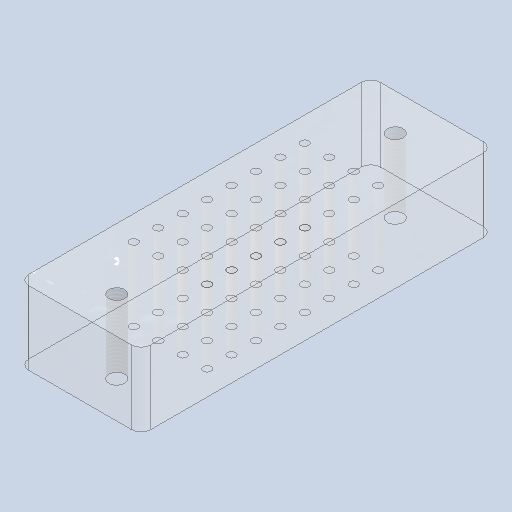
# Autodesk Inventor part: Topo Pressor TL 32
Saved by Autodesk Inventor 2026 (Build 300175050, 175E)
## iProperties
Company: Delta
Created: 2025-06-25
Part Number: Topo Pressor TL 32
Material: Acrílico TP
Document SubType Name: Modeling
Designer: Kedson neves
Density: 1.19 g/cm^3
Appearance: Transparent - Clear
Description: Topo Pressor TL 32
Mass: 30.5078 g
Surface Area: 91.1567 cm^2
Volume: 25.6368 cm^3
Project: FCT
Checked By: William Pinheiro
Dimensões: 15 x 25 x 72
Total: 1
Author: Kedson Neves
Revision Number: 00
Autodesk Inventor part; units mm, degrees
ref_plane "YZ Plane" through (0, 0, 0) normal (1, 0, 0) x (0, 1, 0)
ref_plane "XZ Plane" through (0, 0, 0) normal (0, 1, 0) x (-1, 0, 0)
ref_plane "XY Plane" through (0, 0, 0) normal (0, 0, 1) x (1, 0, 0)
sketch "Sketch1" plane through (0, 0, 0) normal (0, 0, 1) x (1, 0, 0)
  line L0 (-17.5, 0) -> (17.5, 0) construction
  line L1 (0, -50.4) -> (0, 50.4) construction
  line L2 (-12.5, 36) -> (12.5, 36)
  line L3 (12.5, 36) -> (12.5, -36)
  line L4 (12.5, -36) -> (-12.5, -36)
  line L5 (-12.5, -36) -> (-12.5, 36)
  line L6 (-7.5, -17.5) -> (7.5, -17.5) construction
  line L7 (7.5, -17.5) -> (7.5, 17.5) construction
  line L8 (7.5, 17.5) -> (-7.5, 17.5) construction
  line L9 (-7.5, 17.5) -> (-7.5, -17.5) construction
  line L10 (0, 17.5) -> (0, -17.5) construction
  circle A0 centre (0, -28.5) radius 4 construction
  line L11 (-10.5, -20.5) -> (10.5, -20.5) construction
  line L12 (10.5, -20.5) -> (10.5, 20.5) construction
  line L13 (10.5, 20.5) -> (-10.5, 20.5) construction
  line L14 (-10.5, 20.5) -> (-10.5, -20.5) construction
  point P0 (-7.5, -12.5)
  point P1 (-7.5, -7.5)
  point P2 (-7.5, -2.5)
  point P3 (-7.5, 2.5)
  point P4 (-7.5, 7.5)
  point P5 (-7.5, 12.5)
  point P6 (-2.5, -17.5)
  point P7 (-2.5, -12.5)
  point P8 (-2.5, -7.5)
  point P9 (-2.5, -2.5)
  point P10 (-2.5, 2.5)
  point P11 (-2.5, 7.5)
  point P12 (-2.5, 12.5)
  point P13 (-2.5, 17.5)
  point P14 (2.5, -17.5)
  point P15 (2.5, -12.5)
  point P16 (2.5, -7.5)
  point P17 (2.5, -2.5)
  point P18 (2.5, 2.5)
  point P19 (2.5, 7.5)
  point P20 (2.5, 12.5)
  point P21 (2.5, 17.5)
  point P22 (7.5, -12.5)
  point P23 (7.5, -7.5)
  point P24 (7.5, -2.5)
  point P25 (7.5, 2.5)
  point P26 (7.5, 7.5)
  point P27 (7.5, 12.5)
  point P28 (7.5, 17.5)
  point P29 (0, 28.5)
  dimension "d0" = 72
  dimension "d1" = 25
  dimension "d4" = 5
  dimension "d7" = 5
  dimension "d19" = 7.5
  dimension "d20" = 8
  dimension "d21" = 3
  dimension "d22" = 41
  dimension "d23" = 21
  dimension "d39" = 57
  constraints: 24 end point, 6 parallel, 3 horizontal, 3 perpendicular, 2 midpoint, 2 point on line, 1 centre point, 1 coincident, 1 symmetric about line, 1 vertical, 38 other
  measures "d0" distance of L4.end L2.start
  measures "d1" distance of L2.start L2.end
  measures "d4" distance of L6.start point (-7.5, -12.5)
  measures "d7" distance of L6.start point (-2.5, -17.5)
  measures "d19" distance from line of L4 point (0, -28.5)
  measures "d20" diameter of A0
  measures "d21" distance between parallel lines of L14 L9
  measures "d22" distance between parallel lines of L11 L13
  measures "d23" distance between parallel lines of L12 L14
  measures "d39" distance of point (0, 28.5) point (0, -28.5)
extrude "Extrusion1" add sketch "Sketch1" against normal blind 15
hole "Hole1" at (-7.5, -17.5, 0) at (-7.5, -12.5, 0) at (-7.5, -7.5, 0) at (-7.5, -2.5, 0) at (-7.5, 2.5, 0) at (-7.5, 7.5, 0) at (-7.5, 12.5, 0) at (-7.5, 17.5, 0) at (-2.5, -17.5, 0) at (-2.5, -12.5, 0) at (-2.5, -7.5, 0) at (-2.5, -2.5, 0) at (-2.5, 2.5, 0) at (-2.5, 7.5, 0) at (-2.5, 12.5, 0) at (-2.5, 17.5, 0) at (2.5, -17.5, 0) at (2.5, -12.5, 0) at (2.5, -7.5, 0) at (2.5, -2.5, 0) at (2.5, 2.5, 0) at (2.5, 7.5, 0) at (2.5, 12.5, 0) at (2.5, 17.5, 0) at (7.5, -17.5, 0) at (7.5, -12.5, 0) at (7.5, -7.5, 0) at (7.5, -2.5, 0) at (7.5, 2.5, 0) at (7.5, 7.5, 0) at (7.5, 12.5, 0) at (7.5, 17.5, 0) at (7.5, 17.5, 0) direction (0, 0, -1) diameter 1.68 end through all
hole "Hole2" at (0, 28.5, 0) at (0, -28.5, 0) direction (0, 0, -1) diameter 3.242 end through all thread size "M4x0.7" class "6H" standard "ISO Metric profile"
fillet "Fillet1" radius 2 4 edges at (-12.5, -36, -7.5) (12.5, -36, -7.5) (-12.5, 36, -7.5) (12.5, 36, -7.5)
pattern_of_nothing "Rectangular Pattern1"
equation "\"d34\" = d4"
equation "\"d37\" = d7"
body "Solid1"
